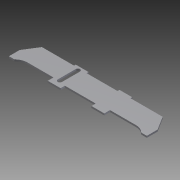
# Autodesk Inventor part: Deslizador
Saved by Autodesk Inventor 2011 (Build 150239000, 239)
## iProperties
Created: 2014-08-04
Part Number: Deslizador
Document SubType Name: Modeling
Designer: amatiasq
Density: 1 g/cm^3
Author: amatiasq
Autodesk Inventor part; units mm, degrees
ref_plane "YZ Plane" through (0, 0, 0) normal (1, 0, 0) x (0, 1, 0)
ref_plane "XZ Plane" through (0, 0, 0) normal (0, 1, 0) x (-1, 0, 0)
ref_plane "XY Plane" through (0, 0, 0) normal (0, 0, 1) x (1, 0, 0)
sketch "Boceto1" plane through (0, 0, 0) normal (0, 0, 1) x (1, 0, 0)
  line L0 (0, 0) -> (18, 0)
  line L1 (18, 0) -> (18, -5)
  line L2 (18, -5) -> (33, -5)
  line L3 (33, -5) -> (33, 1.7)
  line L4 (33, 1.7) -> (64, 1.7)
  arc A0 (74, -2.8) -> (64, 1.7) centre (63.2705, -13.2822) ccw
  line L5 (74, -2.8) -> (80.5, -2.8)
  line L6 (80.5, -2.8) -> (80.5, 9.7)
  line L7 (0, 0) -> (0, 25.4)
  line L8 (0, 25.4) -> (18, 25.4)
  line L9 (18, 25.4) -> (18, 27.7)
  line L10 (18, 27.7) -> (33, 27.7)
  line L11 (33, 27.7) -> (33, 25.7)
  line L12 (33, 25.7) -> (70.5, 25.7)
  line L13 (70.5, 25.7) -> (80.5, 9.7)
  line L14 (0, 0) -> (-18, 0)
  line L15 (-18, 0) -> (-18, -5)
  line L16 (-18, -5) -> (-33, -5)
  line L17 (-33, -5) -> (-33, 1.7)
  line L18 (-33, 1.7) -> (-64, 1.7)
  arc A1 (-64, 1.7) -> (-74, -2.8) centre (-63.2705, -13.2822) ccw
  line L19 (-74, -2.8) -> (-80.5, -2.8)
  line L20 (-80.5, -2.8) -> (-80.5, 9.7)
  line L21 (0, 25.4) -> (-18, 25.4)
  line L22 (-18, 25.4) -> (-18, 27.7)
  line L23 (-18, 27.7) -> (-33, 27.7)
  line L24 (-33, 27.7) -> (-33, 25.7)
  line L25 (-33, 25.7) -> (-70.5, 25.7)
  line L26 (-70.5, 25.7) -> (-80.5, 9.7)
  dimension "d0" = 18
  dimension "d1" = 5
  dimension "d2" = 15
  dimension "d3" = 6.7
  dimension "d4" = 31
  dimension "d5" = 15
  dimension "d6" = 10
  dimension "d7" = 4.5
  dimension "d8" = 6.5
  dimension "d9" = 12.5
  dimension "d12" = 2.3
  dimension "d13" = 15
  dimension "d14" = 2
  dimension "d15" = 37.5
  dimension "d17" = 24
  constraints: 54 end point, 14 symmetric about line, 7 parallel, 6 perpendicular, 4 point on circle, 2 centre point, 1 horizontal, 1 other
  measures "d0" distance of L0.start L0.end
  measures "d1" distance of L0.end L1.end
  measures "d2" distance of L1.end L2.end
  measures "d3" distance of L2.end L3.end
  measures "d4" distance of L3.end L4.end
  measures "d5" radius of A0
  measures "d6" horizontal distance of L5.start L4.end
  measures "d7" vertical distance of L5.start L4.end
  measures "d8" distance of L5.start L5.end
  measures "d9" distance of L5.end L6.end
  measures "d12" distance of L8.end L9.end
  measures "d13" distance of L9.end L10.end
  measures "d14" distance of L10.end L11.end
  measures "d15" distance of L11.end L12.end
  measures "d17" vertical distance of L12.end L4.end
extrude "Extrusión1" add sketch "Boceto1" along normal blind 2
sketch "Boceto2" plane through (0, 0, 2) normal (0, 0, 1) x (1, 0, 0)
  line L0 (-18, 25.4) -> (18, 25.4) projected
  line L1 (-26, 25.7) -> (-26, 25.7)
  line L2 (-23.5, 23.2) -> (-23.5, 2.2)
  line L3 (-26, -0.3) -> (-26, -0.3)
  line L4 (-28.5, 2.2) -> (-28.5, 23.2)
  line L5 (0, 0) -> (0, 25.4)
  line L6 (0, 12.7) -> (-35.7908, 12.7)
  arc A0 (-26, 25.7) -> (-28.5, 23.2) centre (-26, 23.2) ccw
  arc A1 (-23.5, 23.2) -> (-26, 25.7) centre (-26, 23.2) ccw
  arc A2 (-26, -0.3) -> (-23.5, 2.2) centre (-26, 2.2) ccw
  arc A3 (-28.5, 2.2) -> (-26, -0.3) centre (-26, 2.2) ccw
  point P0 (-28.5, 25.7)
  point P1 (-23.5, -0.3)
  point P2 (-23.5, 25.7)
  point P3 (-28.5, -0.3)
  point P4 (-23.5, 12.7)
  dimension "d20" = 23.5
  dimension "d21" = 5
  dimension "d22" = 26
  dimension "d24" = 2.5
  constraints: 12 end point, 9 point on line, 8 point on circle, 8 tangent, 4 centre point, 3 equal radius, 3 midpoint, 2 parallel, 2 perpendicular, 1 horizontal
  measures "d20" horizontal distance of L5.start point (-23.5, -0.3)
  measures "d21" distance of point (-28.5, 25.7) point (-23.5, 25.7)
  measures "d22" distance of point (-28.5, -0.3) point (-28.5, 25.7)
  measures "d24" radius of A0
extrude "Extrusión2" cut sketch "Boceto2" against normal through all
